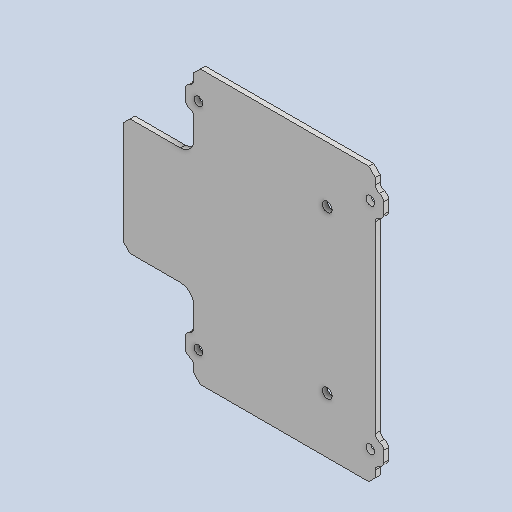
# Autodesk Inventor part: power_board
Saved by Autodesk Inventor 2025 (Build 290162000, 162)
## iProperties
Created: 2026-08-11
Part Number: power_board
Material: Типовые
Document SubType Name: Modeling
Designer: garin
Density: 1 g/cm^3
Appearance: По умолчанию
Author: garin
Autodesk Inventor part; units mm, degrees
ref_plane "YZ Plane" through (0, 0, 0) normal (1, 0, 0) x (0, 1, 0)
ref_plane "XZ Plane" through (0, 0, 0) normal (0, 1, 0) x (-1, 0, 0)
ref_plane "XY Plane" through (0, 0, 0) normal (0, 0, 1) x (1, 0, 0)
sketch "Эскиз1" plane through (0, 0, 0) normal (0, 0, 1) x (1, 0, 0)
  line L0 (-30, 41.5) -> (28, 41.5)
  line L1 (30, 39.5) -> (30, -39.5)
  line L2 (28, -41.5) -> (-30, -41.5)
  line L3 (-30, -41.5) -> (-30, 41.5)
  line L4 (-30, 41.5) -> (30, -41.5) construction
  line L5 (30, 41.5) -> (-30, -41.5) construction
  line L6 (-30, -41.5) -> (-42.5, -41.5)
  line L7 (-46.5, -37.5) -> (-46.5, 37.5)
  line L8 (-42.5, 41.5) -> (-30, 41.5)
  line L9 (-30, 41.5) -> (-30, -41.5)
  line L10 (-42.5, -41.5) -> (-46.5, -37.5)
  line L11 (-46.5, 37.5) -> (-42.5, 41.5)
  line L12 (28, 41.5) -> (30, 39.5)
  line L13 (28, -41.5) -> (30, -39.5)
  line L14 (0, 0) -> (-23.984, 0) construction
  line L15 (-23.984, 0) -> (-23.984, 15.7) construction
  line L16 (-23.984, 15.7) -> (0, 15.7) construction
  line L17 (0, 15.7) -> (0, 0) construction
  circle A0 centre (-23.984, 15.7) radius 1.6
  circle A1 centre (-23.984, -15.7) radius 1.6
  circle A2 centre (23.984, 15.7) radius 1.6
  circle A3 centre (23.984, -15.7) radius 1.6
  line L18 (-46.5, -41.5) -> (-25.168, -41.5)
  line L19 (-25.168, -41.5) -> (-25.168, -21.7)
  line L20 (-29.168, -17.7) -> (-46.5, -17.7)
  line L21 (-46.5, -17.7) -> (-46.5, -41.5)
  arc A4 (-25.168, -21.7) -> (-29.168, -17.7) centre (-29.168, -21.7) ccw
  line L22 (-25.168, 41.5) -> (-25.168, 21.7)
  line L23 (-29.168, 17.7) -> (-46.5, 17.7)
  arc A5 (-29.168, 17.7) -> (-25.168, 21.7) centre (-29.168, 21.7) ccw
  point P0 (-46.5, 41.5)
  point P1 (-25.168, -17.7)
  point P2 (-25.168, 41.5)
  point P3 (-46.5, -17.7)
  point P4 (-25.168, -41.5)
  dimension "d0" = 60
  dimension "d1" = 83
  dimension "d2" = 16.5
  dimension "d3" = 83
  dimension "d6" = 4
  dimension "d7" = 4
  dimension "d8" = 4
  dimension "d9" = 4
  dimension "d10" = 2
  dimension "d11" = 2
  dimension "d12" = 2
  dimension "d13" = 2
  dimension "d14" = 23.984
  dimension "d15" = 15.7
  dimension "d16" = 3.2
  dimension "d17" = 21.332
  dimension "d18" = 23.8
  dimension "d19" = 4
  constraints: 48 end point, 10 point on line, 8 parallel, 8 symmetric about line, 6 centre point, 4 horizontal, 4 perpendicular, 4 point on circle, 2 midpoint, 2 tangent, 1 coincident, 4 other
  measures "d0" distance of L4.end L2.end
  measures "d1" distance of L5.start L4.end
  measures "d2" distance of point (-46.5, 41.5) L8.end
  measures "d3" distance of L18.start point (-46.5, 41.5)
  measures "d6" distance of L6.end L18.start
  measures "d7" distance of L7.start L18.start
  measures "d8" distance of L7.end point (-46.5, 41.5)
  measures "d9" distance of L8.start point (-46.5, 41.5)
  measures "d10" distance of L0.end L5.start
  measures "d11" distance of L1.start L5.start
  measures "d12" distance of L2.start L4.end
  measures "d13" distance of L1.end L4.end
  measures "d14" distance of L15.end L16.end
  measures "d15" distance of L14.end L15.end
  measures "d16" diameter of A0
  measures "d17" distance of L20.end point (-25.168, -17.7)
  measures "d18" distance of point (-25.168, -17.7) L18.end
  measures "d19" radius of A4
extrude "Выдавливание1" add sketch "Эскиз1" along normal blind 1.5 contours L0 L12 L1 L13 L2 L19 A4 L20 L3 L23 A5 L22 | L3 L20 L7 L23 | A0 | A1 | A2 | A3
chamfer "Фаска1" distance 2 angle 45 4 edges at (-46.5, -17.7, 0.75) (-46.5, 17.7, 0.75) (-25.168, -41.5, 0.75) (-25.168, 41.5, 0.75)
sketch "Эскиз2" plane through (0, 0, 0) normal (0, 0, -1) x (-1, 0, 0)
  arc A0 (43.584, 19.7) -> (47.584, 23.7) centre (43.584, 23.7) ccw projected
  arc A1 (27.668, 34.3) -> (26.418, 35.8612) centre (26.068, 34.3) ccw projected
  line L0 (27.668, 34.3) -> (27.668, 31.0225) projected
  arc A2 (26.418, 29.4612) -> (27.668, 31.0225) centre (26.068, 31.0225) ccw projected
  arc A3 (26.418, 29.4612) -> (25.168, 27.9) centre (26.768, 27.9) ccw projected
  line L1 (25.168, 27.9) -> (25.168, 23.7) projected
  arc A4 (25.168, 23.7) -> (29.168, 19.7) centre (29.168, 23.7) ccw projected
  line L2 (29.168, 19.7) -> (43.584, 19.7) projected
  arc A5 (43.584, 19.7) -> (47.584, 23.7) centre (43.584, 23.7) ccw projected
  line L3 (47.584, 23.7) -> (47.584, 39.2) projected
  line L4 (47.584, 39.2) -> (25.168, 39.2) projected
  line L5 (25.168, 39.2) -> (25.168, 37.4225) projected
  arc A6 (25.168, 37.4225) -> (26.418, 35.8612) centre (26.768, 37.4225) ccw projected
  line L6 (52.084, -4) -> (58.0913, -4) projected
  line L7 (58.0913, -4) -> (58.0913, -38.5) projected
  line L8 (58.0913, -38.5) -> (69.3773, -38.5) projected
  line L9 (69.3773, -38.5) -> (69.3773, 32.5) projected
  line L10 (69.3773, 32.5) -> (58.0913, 32.5) projected
  line L11 (58.0913, 32.5) -> (58.0913, 24) projected
  line L12 (58.0913, 24) -> (52.084, 24) projected
  line L13 (52.084, 24) -> (52.084, 13.5) projected
  line L14 (52.084, 13.5) -> (34.584, 13.5) projected
  arc A7 (34.584, 13.5) -> (34.584, 1.5) centre (34.584, 7.5) ccw projected
  line L15 (34.584, 1.5) -> (47.084, 1.5) projected
  line L16 (47.084, 1.5) -> (47.084, -3.7639) projected
  spline S0 degree 3 poles (48.084, -6) (47.8036, -5.6035) (47.4716, -5.1246) (47.1717, -4.4032) (47.084, -4.0595) (47.084, -3.7639) knots 0.566831 0.566831 0.566831 0.566831 0.71252 0.71252 0.801197 0.801197 0.801197 0.801197 projected
  line L17 (51.084, -6) -> (48.084, -6) projected
  spline S1 degree 3 poles (52.084, -3.7639) (52.084, -4.0595) (51.9963, -4.4032) (51.6964, -5.1246) (51.3644, -5.6035) (51.084, -6) knots 0 0 0 0 0.088677 0.088677 0.234365 0.234365 0.234365 0.234365 projected
  line L18 (52.084, -3.7639) -> (52.084, -4) projected
  line L19 (74.484, -42.6) -> (-79.316, -42.6) projected
  line L20 (-79.316, -42.6) -> (-79.316, 42.6) projected
  line L21 (6.584, 42.6) -> (74.484, 42.6) projected
  line L22 (74.484, 42.6) -> (74.484, -42.6) projected
  circle A8 centre (23.684, -32.7) radius 1.6 projected
  circle A9 centre (23.684, 32.7) radius 1.6 projected
  line L23 (20.484, 41.2) -> (6.584, 41.2) projected
  line L24 (-25.316, 41.2) -> (-25.316, -41.2) projected
  line L25 (-25.316, -41.2) -> (20.484, -41.2) projected
  line L26 (20.484, -41.2) -> (20.484, 41.2) projected
  circle A10 centre (-28.516, -32.7) radius 1.6 projected
  circle A11 centre (-28.516, 32.7) radius 1.6 projected
  arc A12 (-32.5, 31.0225) -> (-31.25, 29.4612) centre (-30.9, 31.0225) ccw projected
  line L27 (-32.5, 31.0225) -> (-32.5, 34.3775) projected
  arc A13 (-31.25, 35.9388) -> (-32.5, 34.3775) centre (-30.9, 34.3775) ccw projected
  arc A14 (-31.25, 35.9388) -> (-30, 37.5) centre (-31.6, 37.5) ccw projected
  line L28 (-30, 37.5) -> (-30, 39.2) projected
  line L29 (-30, 39.2) -> (-52.416, 39.2) projected
  line L30 (-52.416, 39.2) -> (-52.416, 23.7) projected
  arc A15 (-52.416, 23.7) -> (-48.416, 19.7) centre (-48.416, 23.7) ccw projected
  line L31 (-48.416, 19.7) -> (-34, 19.7) projected
  arc A16 (-34, 19.7) -> (-30, 23.7) centre (-34, 23.7) ccw projected
  line L32 (-30, 23.7) -> (-30, 27.9) projected
  arc A17 (-30, 27.9) -> (-31.25, 29.4612) centre (-31.6, 27.9) ccw projected
  arc A18 (-32.5, -34.3) -> (-31.25, -35.8612) centre (-30.9, -34.3) ccw projected
  line L33 (-32.5, -34.3) -> (-32.5, -31.0225) projected
  arc A19 (-31.25, -29.4612) -> (-32.5, -31.0225) centre (-30.9, -31.0225) ccw projected
  arc A20 (-31.25, -29.4612) -> (-30, -27.9) centre (-31.6, -27.9) ccw projected
  line L34 (-30, -27.9) -> (-30, -23.7) projected
  arc A21 (-30, -23.7) -> (-34, -19.7) centre (-34, -23.7) ccw projected
  line L35 (-34, -19.7) -> (-48.416, -19.7) projected
  arc A22 (-48.416, -19.7) -> (-52.416, -23.7) centre (-48.416, -23.7) ccw projected
  line L36 (-52.416, -23.7) -> (-52.416, -39.2) projected
  line L37 (-52.416, -39.2) -> (-30, -39.2) projected
  line L38 (-30, -39.2) -> (-30, -37.4225) projected
  arc A23 (-30, -37.4225) -> (-31.25, -35.8612) centre (-31.6, -37.4225) ccw projected
  arc A24 (26.418, -35.9388) -> (27.668, -34.3775) centre (26.068, -34.3775) ccw projected
  arc A25 (26.418, -35.9388) -> (25.168, -37.5) centre (26.768, -37.5) ccw projected
  line L39 (25.168, -37.5) -> (25.168, -39.2) projected
  line L40 (25.168, -39.2) -> (47.584, -39.2) projected
  line L41 (47.584, -39.2) -> (47.584, -23.7) projected
  arc A26 (47.584, -23.7) -> (43.584, -19.7) centre (43.584, -23.7) ccw projected
  line L42 (43.584, -19.7) -> (29.168, -19.7) projected
  arc A27 (29.168, -19.7) -> (25.168, -21.7) centre (29.168, -23.7) ccw projected
  line L43 (25.168, -21.7) -> (25.168, -27.9) projected
  arc A28 (25.168, -27.9) -> (26.418, -29.4612) centre (26.768, -27.9) ccw projected
  arc A29 (27.668, -31.0225) -> (26.418, -29.4612) centre (26.068, -31.0225) ccw projected
  line L44 (27.668, -31.0225) -> (27.668, -34.3775) projected
  line L45 (25.168, -39.2) -> (25.168, 39.2)
  line L46 (25.168, -21.7) -> (25.168, -39.5) projected
  line L47 (-30, 39.2) -> (-30, -39.2)
  line L48 (-11.416, 42.6) -> (-11.416, 41.2) projected
  line L49 (-11.416, 41.2) -> (-25.316, 41.2) projected
  line L50 (6.584, 41.2) -> (6.584, 42.6) projected
  line L51 (-79.316, 42.6) -> (-11.416, 42.6) projected
  point P0 (0, 0)
  point P1 (-30, -37.4225)
  point P2 (-30, -27.9)
  point P3 (-30, 27.9)
  point P4 (-30, 37.5)
  point P5 (25.168, 37.4225)
  point P6 (25.168, 27.9)
  point P7 (25.168, -37.5)
  point P8 (25.168, -27.9)
  constraints: 4 end point, 2 collinear, 1 other
extrude "Выдавливание2" add sketch "Эскиз2" against normal blind 1.5 contours L45 A9 A6 A1 L0 A2 A3 | L45 A9 | A28 A29 L44 A24 A25 L45 A8 | A8 L45 | L47 A10 | A10 L47 A23 A18 L33 A19 A20 | A17 A12 L27 A13 A14 L47 A11 | A11 L47 picked at (25.1894, 32.5653) picked at (25.1894, -32.5653) picked at (-30.0289, -32.5985) picked at (-30.0289, 32.8015)
sketch "Эскиз3" plane through (0, 0, 0) normal (0, 0, -1) x (-1, 0, 0)
  arc A0 (27.668, 34.3) -> (26.418, 35.8612) centre (26.068, 34.3) ccw projected
  line L0 (27.668, 34.3) -> (27.668, 31.0225) projected
  arc A1 (26.418, 29.4612) -> (27.668, 31.0225) centre (26.068, 31.0225) ccw projected
  arc A2 (26.418, 29.4612) -> (25.168, 27.9) centre (26.768, 27.9) ccw projected
  line L1 (25.168, 27.9) -> (25.168, 23.7) projected
  arc A3 (25.168, 23.7) -> (29.168, 19.7) centre (29.168, 23.7) ccw projected
  line L2 (29.168, 19.7) -> (43.584, 19.7) projected
  arc A4 (43.584, 19.7) -> (47.584, 23.7) centre (43.584, 23.7) ccw projected
  line L3 (47.584, 23.7) -> (47.584, 39.2) projected
  line L4 (47.584, 39.2) -> (25.168, 39.2) projected
  line L5 (25.168, 39.2) -> (25.168, 37.4225) projected
  arc A5 (25.168, 37.4225) -> (26.418, 35.8612) centre (26.768, 37.4225) ccw projected
  line L6 (52.084, -4) -> (58.0913, -4) projected
  line L7 (58.0913, -4) -> (58.0913, -38.5) projected
  line L8 (58.0913, -38.5) -> (69.3773, -38.5) projected
  line L9 (69.3773, -38.5) -> (69.3773, 32.5) projected
  line L10 (69.3773, 32.5) -> (58.0913, 32.5) projected
  line L11 (58.0913, 32.5) -> (58.0913, 24) projected
  line L12 (58.0913, 24) -> (52.084, 24) projected
  line L13 (52.084, 24) -> (52.084, 13.5) projected
  line L14 (52.084, 13.5) -> (34.584, 13.5) projected
  arc A6 (34.584, 13.5) -> (34.584, 1.5) centre (34.584, 7.5) ccw projected
  line L15 (34.584, 1.5) -> (47.084, 1.5) projected
  line L16 (47.084, 1.5) -> (47.084, -3.7639) projected
  spline S0 degree 3 poles (48.084, -6) (47.8036, -5.6035) (47.4716, -5.1246) (47.1717, -4.4032) (47.084, -4.0595) (47.084, -3.7639) knots 0.566831 0.566831 0.566831 0.566831 0.71252 0.71252 0.801197 0.801197 0.801197 0.801197 projected
  line L17 (51.084, -6) -> (48.084, -6) projected
  spline S1 degree 3 poles (52.084, -3.7639) (52.084, -4.0595) (51.9963, -4.4032) (51.6964, -5.1246) (51.3644, -5.6035) (51.084, -6) knots 0 0 0 0 0.088677 0.088677 0.234365 0.234365 0.234365 0.234365 projected
  line L18 (52.084, -3.7639) -> (52.084, -4) projected
  line L19 (74.484, -42.6) -> (-79.316, -42.6) projected
  line L20 (-79.316, -42.6) -> (-79.316, 42.6) projected
  line L21 (6.584, 42.6) -> (74.484, 42.6) projected
  line L22 (74.484, 42.6) -> (74.484, -42.6) projected
  circle A7 centre (23.684, -32.7) radius 1.6 projected
  circle A8 centre (23.684, 32.7) radius 1.6 projected
  line L23 (20.484, 41.2) -> (6.584, 41.2) projected
  line L24 (-25.316, 41.2) -> (-25.316, -41.2) projected
  line L25 (-25.316, -41.2) -> (20.484, -41.2) projected
  line L26 (20.484, -41.2) -> (20.484, 41.2) projected
  circle A9 centre (-28.516, -32.7) radius 1.6 projected
  circle A10 centre (-28.516, 32.7) radius 1.6 projected
  arc A11 (-32.5, 31.0225) -> (-31.25, 29.4612) centre (-30.9, 31.0225) ccw projected
  line L27 (-32.5, 31.0225) -> (-32.5, 34.3775) projected
  arc A12 (-31.25, 35.9388) -> (-32.5, 34.3775) centre (-30.9, 34.3775) ccw projected
  arc A13 (-31.25, 35.9388) -> (-30, 37.5) centre (-31.6, 37.5) ccw projected
  line L28 (-30, 37.5) -> (-30, 39.2) projected
  line L29 (-30, 39.2) -> (-52.416, 39.2) projected
  line L30 (-52.416, 39.2) -> (-52.416, 23.7) projected
  arc A14 (-52.416, 23.7) -> (-48.416, 19.7) centre (-48.416, 23.7) ccw projected
  line L31 (-48.416, 19.7) -> (-34, 19.7) projected
  arc A15 (-34, 19.7) -> (-30, 23.7) centre (-34, 23.7) ccw projected
  line L32 (-30, 23.7) -> (-30, 27.9) projected
  arc A16 (-30, 27.9) -> (-31.25, 29.4612) centre (-31.6, 27.9) ccw projected
  arc A17 (-32.5, -34.3) -> (-31.25, -35.8612) centre (-30.9, -34.3) ccw projected
  line L33 (-32.5, -34.3) -> (-32.5, -31.0225) projected
  arc A18 (-31.25, -29.4612) -> (-32.5, -31.0225) centre (-30.9, -31.0225) ccw projected
  arc A19 (-31.25, -29.4612) -> (-30, -27.9) centre (-31.6, -27.9) ccw projected
  line L34 (-30, -27.9) -> (-30, -23.7) projected
  arc A20 (-30, -23.7) -> (-34, -19.7) centre (-34, -23.7) ccw projected
  line L35 (-34, -19.7) -> (-48.416, -19.7) projected
  arc A21 (-48.416, -19.7) -> (-52.416, -23.7) centre (-48.416, -23.7) ccw projected
  line L36 (-52.416, -23.7) -> (-52.416, -39.2) projected
  line L37 (-52.416, -39.2) -> (-30, -39.2) projected
  line L38 (-30, -39.2) -> (-30, -37.4225) projected
  arc A22 (-30, -37.4225) -> (-31.25, -35.8612) centre (-31.6, -37.4225) ccw projected
  arc A23 (26.418, -35.9388) -> (27.668, -34.3775) centre (26.068, -34.3775) ccw projected
  arc A24 (26.418, -35.9388) -> (25.168, -37.5) centre (26.768, -37.5) ccw projected
  line L39 (25.168, -37.5) -> (25.168, -39.2) projected
  line L40 (25.168, -39.2) -> (47.584, -39.2) projected
  line L41 (47.584, -39.2) -> (47.584, -23.7) projected
  arc A25 (47.584, -23.7) -> (43.584, -19.7) centre (43.584, -23.7) ccw projected
  line L42 (43.584, -19.7) -> (29.168, -19.7) projected
  arc A26 (29.168, -19.7) -> (25.168, -23.7) centre (29.168, -23.7) ccw projected
  line L43 (25.168, -23.7) -> (25.168, -27.9) projected
  arc A27 (25.168, -27.9) -> (26.418, -29.4612) centre (26.768, -27.9) ccw projected
  arc A28 (27.668, -31.0225) -> (26.418, -29.4612) centre (26.068, -31.0225) ccw projected
  line L44 (27.668, -31.0225) -> (27.668, -34.3775) projected
  line L45 (25.168, -39.5) -> (23.168, -41.5) projected
  line L46 (23.168, -41.5) -> (25.168, -41.5) construction
  line L47 (25.168, -41.5) -> (25.168, -39.5) construction
  line L48 (25.168, -39.5) -> (23.168, -39.5) construction
  line L49 (23.168, -39.5) -> (23.168, -41.5) construction
  line L50 (25.168, -41.5) -> (-15.416, -41.5) construction
  line L51 (-15.416, -41.5) -> (-15.416, -24.5) construction
  line L52 (-15.416, -24.5) -> (25.168, -24.5) construction
  line L53 (25.168, -24.5) -> (25.168, -41.5) construction
  circle A29 centre (-15.416, -24.5) radius 1.5
  line L54 (-25.316, 0) -> (20.484, 0) construction
  circle A30 centre (-15.416, 24.5) radius 1.5
  circle A31 centre (23.684, -32.7) radius 1.35
  circle A32 centre (-28.516, -32.7) radius 1.35
  circle A33 centre (-28.516, 32.7) radius 1.35
  circle A34 centre (23.684, 32.7) radius 1.35
  line L55 (-11.416, 42.6) -> (-11.416, 41.2) projected
  line L56 (-11.416, 41.2) -> (-25.316, 41.2) projected
  line L57 (6.584, 41.2) -> (6.584, 42.6) projected
  line L58 (-79.316, 42.6) -> (-11.416, 42.6) projected
  point P0 (0, 0)
  dimension "d25" = 40.584
  dimension "d26" = 17
  dimension "d27" = 3
  dimension "d28" = 2.7
  dimension "d29" = 2.7
  dimension "d30" = 2.7
  dimension "d31" = 2.7
  constraints: 18 end point, 6 centre point, 5 coincident, 4 parallel, 2 horizontal, 2 midpoint, 2 perpendicular, 1 symmetric about line, 1 other
  measures "d25" distance of L51.end L52.end
  measures "d26" distance of L50.end L51.end
  measures "d27" diameter of A29
  measures "d28" diameter of A31
  measures "d29" diameter of A32
  measures "d30" diameter of A33
  measures "d31" diameter of A34
extrude "Выдавливание3" cut sketch "Эскиз3" against normal blind 1.5 contours A29 | A30 | A31 | A32 | A33 | A34
equation "\"d7\" = d6"
equation "\"d9\" = d8"
equation "\"d11\" = d10"
